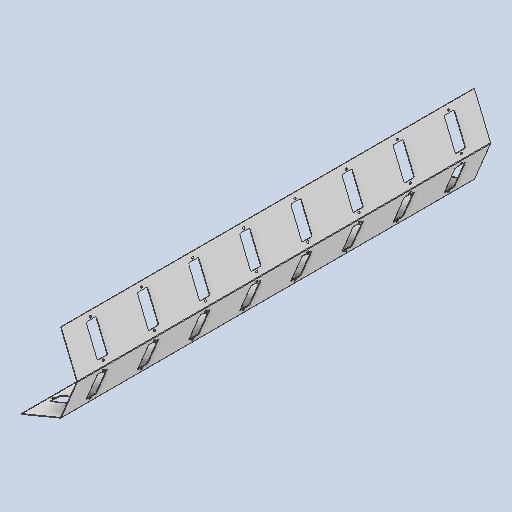
# Autodesk Inventor part: ДМС 100 Барабан Лист №1
Saved by Autodesk Inventor 2024.2 (Build 282272000, 272)
## iProperties
Created: 2024-04-28
Part Number: ДМС 100 Барабан Лист №1
Material: Generic
Document SubType Name: Sheet Metal
Designer: pokla
Density: 1 g/cm^3
Appearance: Default
Sheet Metal Rule: Default
Author: pokla
Autodesk Inventor part; units mm, degrees
ref_plane "YZ Plane" through (0, 0, 0) normal (1, 0, 0) x (0, 1, 0)
ref_plane "XZ Plane" through (0, 0, 0) normal (0, 1, 0) x (-1, 0, 0)
ref_plane "XY Plane" through (0, 0, 0) normal (0, 0, 1) x (1, 0, 0)
sketch "Sketch2" plane through (0, 0, 0) normal (0, 0, 1) x (1, 0, 0)
  line L0 (0, 273.845227) -> (193.637817, 193.637817) construction
  line L1 (193.637817, 193.637817) -> (273.845227, 0) construction
  line L2 (273.845227, 0) -> (193.637817, -193.637817) construction
  line L3 (193.637817, -193.637817) -> (0, -273.845227) construction
  line L4 (0, -273.845227) -> (-193.637817, -193.637817) construction
  line L5 (-193.637817, -193.637817) -> (-273.845227, 0) construction
  line L6 (-273.845227, 0) -> (-193.637817, 193.637817) construction
  line L7 (-193.637817, 193.637817) -> (0, 273.845227) construction
  line L8 (194.0205, 192.713937) -> (272.894151, 2.296101)
  line L9 (272.894151, -2.296101) -> (194.588893, -191.341716)
  arc A0 (272.894151, -2.296101) -> (272.894151, 2.296101) centre (267.350873, 0) ccw
  line L10 (191.341716, -194.588893) -> (0.92388, -273.462543)
  arc A1 (191.341716, -194.588893) -> (194.588893, -191.341716) centre (189.045616, -189.045616) ccw
  point P0 (0, 0)
  point P1 (0, 0)
  dimension "d56" = 506
  dimension "d58" = 6
  dimension "d69" = 1
  dimension "d70" = 6
  dimension "d71" = 1
  measures "d56" distance between parallel lines of L6 L2
  measures "d58" radius of A0
  measures "d69" distance of L3.end L10.end
  measures "d70" radius of A1
  measures "d71" distance of L0.end L8.start
contour flange "Contour Flange2" sketch "Sketch2" thickness 3 bend radius 3 width 2020 along (0, 0, -1) mid plane no both sides no wall seen from (233.457325, 97.505019, 0) lies toward (-0.9238795, -0.3826834, 0) curves L8 A0 L9 A1 L10
bend "Bend2"
corner "Corner2"
sketch "Sketch10" plane through (194.588893, -191.341716, 0) normal (0.9238795, -0.3826834, 0) x (0, 0, -1)
  line L0 (1110, 174.81075) -> (1160, 174.81075)
  line L1 (1160, 174.81075) -> (1160, 29.81075)
  line L2 (1160, 29.81075) -> (1110, 29.81075)
  line L3 (1110, 29.81075) -> (1110, 174.81075)
  circle A0 centre (1135, 184.81075) radius 5
  circle A1 centre (1135, 19.81075) radius 5
  line L4 (1110, 102.31075) -> (1160, 102.31075) construction
  line L5 (2020, 204.6215) -> (2020, 0) construction
  line L6 (2020, 204.6215) -> (0, 204.6215) construction
  point P0 (0, 102.31075)
  point P1 (1135, 174.81075)
  point P2 (2020, 102.31075)
  point P3 (1010, 204.6215)
  point P4 (1010, 204.6215)
  dimension "d107" = 145
  dimension "d108" = 50
  dimension "d109" = 10
  dimension "d110" = 10
  dimension "d118" = 125
  constraints: 10 end point, 6 midpoint, 2 centre point, 2 parallel, 1 horizontal, 1 horizontal alignment, 1 perpendicular, 1 vertical alignment, 1 other
  measures "d107" distance of L0.end L1.end
  measures "d108" distance of L0.start L0.end
  measures "d109" diameter of A0
  measures "d110" distance from line of L0 A0.centre
  measures "d118" horizontal distance of point (1010, 204.621) point (1135, 174.811)
extrude "Extrusion4" cut sketch "Sketch10" against normal up to surface (3 mm away)
fillet "Fillet1" radius 5 4 edges at (260.1003, -29.2636, -1160) (260.1003, -29.2636, -1110) (204.6112, -163.2261, -1110) (204.6112, -163.2261, -1160)
pattern_circular "Circular Pattern1" count 3 over 90 about axis through (0, 0, -10) along (0, 0, 1) of "Extrusion4", "Fillet1" both ways yes
pattern_linear "Rectangular Pattern2" count 8 spacing 250 along (0, 0, 1) of "Extrusion4", "Fillet1", "Circular Pattern1" first direction both ways yes
equation "\"d118\" = Отступ_окна_от_середины"
equation "\"d56\" = Барабан_габарит_по_кассетам"
equation "\"d58\" = BendRadius + Thickness"
equation "\"d70\" = BendRadius + Thickness"
equation "\"d107\" = Длина_окна_барабан"
equation "\"d108\" = Ширина_окна_барабан"
equation "\"d109\" = Диам_шпильки_под_кассету"
equation "\"d25\" = Thickness"
equation "\"d26\" = BendReliefWidth"
equation "\"d27\" = BendReliefDepth"
equation "\"d28\" = MinimumRemnant"
equation "\"d29\" = TransitionRadius"
equation "\"d30\" = Барабан_длина_листа"
equation "\"d31\" = BendRadius"
equation "\"d33\" = CornerReliefSize"
equation "\"d34\" = GapSize"
equation "\"d35\" = JacobiRadiusSize"
equation "\"BendRadius\" = Thickness"
equation "\"BendReliefWidth\" = Thickness"
equation "\"BendReliefDepth\" = 0.5 * Thickness"
equation "\"CornerReliefSize\" = 4 * Thickness"
equation "\"MinimumRemnant\" = 2 * Thickness"
equation "\"TransitionRadius\" = BendRadius"
equation "\"JacobiRadiusSize\" = BendRadius"
equation "\"GapSize\" = Thickness"
equation "\"Барабан_габарит_по_кассетам\" = 506"
equation "\"Thickness\" = 3"
equation "\"Длина_окна_барабан\" = 145"
equation "\"Ширина_окна_барабан\" = 50"
equation "\"Диам_шпильки_под_кассету\" = 10"
equation "\"Барабан_длина_листа\" = 2020"
equation "\"Отступ_окна_от_середины\" = 125"
body "Solid2"
